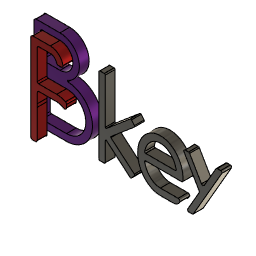
bfkey (Autodesk Fusion 360 design; units mm, degrees)
Autodesk Fusion 360 part; units mm, degrees
sketch "Sketch1" plane through (0, 0, 0) normal (0, 1, 0) x (1, 0, 0)
  line L0 (10, -10) -> (20, -10)
  line L1 (20, -10) -> (20, -150)
  line L2 (20, -150) -> (10, -150)
  line L3 (10, -150) -> (10, -10)
  circle A0 centre (50, -120) radius 30
  circle A1 centre (59.9048, -50.3504) radius 40.3504
  line L4 (20, -150) -> (50, -150)
  line L5 (20, -10) -> (59.9048, -10)
  constraint horizontal L0
  constraint vertical L1
  constraint horizontal L2
  constraint vertical L3
  constraint tangent L1 A0
  constraint coincident A0 L4.end
  constraint tangent A0 L4
  constraint perpendicular L1 L4
  constraint coincident A1 L5.end
  constraint tangent A1 L5
  constraint perpendicular L1 L5
  constraint tangent A0 A1
extrude "Extrude1" add sketch "Sketch1" along normal blind 15 makes body 1
sketch "Sketch2" plane through (0, 0, 0) normal (0, -1, 0) x (1, 0, 0)
  line L0 (50, 150) -> (10, 150)
  line L1 (10, 150) -> (10, 10)
  line L2 (10, 10) -> (59.9048, 10)
  arc A0 (59.9048, 10) -> (54.2238, 90.2988) centre (59.9048, 50.3504) ccw
  arc A1 (54.2238, 90.2988) -> (50, 150) centre (50, 120) ccw
  circle A2 centre (50, 120) radius 20
  line L3 (20, 140) -> (50, 140)
  line L4 (50, 140) -> (50, 100)
  line L5 (50, 100) -> (20, 100)
  line L6 (20, 100) -> (20, 140)
  circle A3 centre (59.9048, 50.3504) radius 30
  line L7 (60.0309, 20.3506) -> (60.0309, 80.3501)
  line L8 (60.0309, 80.3501) -> (20, 80.3501)
  line L9 (20, 80.3501) -> (20, 20.3506)
  line L10 (20, 20.3506) -> (60.0309, 20.3506)
  dimension "d3" = 60
  constraint concentric A1 A2
  constraint horizontal L3
  constraint vertical L4
  constraint horizontal L5
  constraint vertical L6
  constraint coincident A2 L4.end
  constraint concentric A0 A3
  constraint perpendicular L7 L8
  constraint parallel L7 L9
  constraint parallel L8 L10
  constraint coincident A3 L7.end
  constraint vertical L7
  constraint coincident A3 L7.start
  measures "d3" diameter of A3
extrude "Extrude2" cut sketch "Sketch2" against normal blind 50 contours A2 L4 | A2 L4 | A2 L3 L5 L6 | A3 L7 | L7 L8 L9 L10 bodies 1
sketch "Sketch3" plane through (0, 0, 0) normal (0, -1, 0) x (1, 0, 0)
  line L0 (20, 140) -> (50, 140)
  arc A0 (50, 100) -> (50, 140) centre (50, 120) ccw
  line L1 (50, 100) -> (20, 100)
  line L2 (20, 100) -> (20, 140)
  arc A1 (60.0309, 20.3506) -> (60.0309, 80.3501) centre (59.9048, 50.3504) ccw
  line L3 (60.0309, 20.3506) -> (20, 20.3506)
  line L4 (20, 20.3506) -> (20, 80.3501)
  line L5 (20, 80.3501) -> (60.0309, 80.3501)
  line L6 (50, 150) -> (10, 150)
  line L7 (10, 150) -> (10, 10)
  line L8 (10, 10) -> (59.9048, 10)
  arc A2 (59.9048, 10) -> (54.2238, 90.2988) centre (59.9048, 50.3504) ccw
  arc A3 (54.2238, 90.2988) -> (50, 150) centre (50, 120) ccw
  line L9 (20, 0.7007) -> (30, 0.7007)
  line L10 (30, 0.7007) -> (30, 140)
  line L11 (30, 140) -> (20, 140)
  line L12 (20, 140) -> (20, 0.7007)
  line L13 (30, 130) -> (50, 130)
  line L14 (50, 130) -> (50, 140)
  line L15 (50, 140) -> (30, 140)
  line L16 (30, 140) -> (30, 130)
  circle A4 centre (50, 120) radius 20
  circle A5 centre (50, 120) radius 10
  line L17 (60, 120) -> (70, 120)
  circle A6 centre (59.9048, 50.3504) radius 30
  circle A7 centre (59.9048, 50.3504) radius 20
  line L18 (30, 70.3504) -> (60.0309, 70.3504)
  line L19 (60.0309, 70.3504) -> (60.0309, 80.3501)
  line L20 (60.0309, 80.3501) -> (30, 80.3501)
  line L21 (30, 80.3501) -> (30, 70.3504)
  line L22 (75.1346, 63.3138) -> (75.1346, 79.1838)
  dimension "d6" = 40
  constraint horizontal L9
  constraint vertical L10
  constraint horizontal L11
  constraint vertical L12
  constraint coincident L0 L10.end
  constraint horizontal L13
  constraint vertical L14
  constraint horizontal L15
  constraint vertical L16
  constraint coincident L0.end A0.end
  constraint coincident L10 L13.start
  constraint concentric A0 A4
  constraint concentric A4 A5
  constraint coincident L13.end A5
  constraint coincident A5 L17.start
  constraint midpoint A0 L17.end
  constraint horizontal L17
  constraint concentric A1 A6
  constraint coincident A1.end A6
  constraint concentric A1 A7
  constraint horizontal L18
  constraint vertical L19
  constraint horizontal L20
  constraint vertical L21
  constraint coincident A1.end L5.end
  constraint midpoint L10 L18.start
  constraint coincident A7 L22.start
  constraint vertical L22
  constraint tangent A7 L18
  measures "d6" diameter of A7
extrude "Extrude3" add sketch "Sketch3" along normal blind 15 separate body contours A6 L18 L19 | L0 L1 L2 L10 L11 L12 L16 | L0 L10 L13 L15 L16 A4 | L1 L5 L10 L12 | A0 L14 A4 A5 L17 | L13 L14 A4 | L3 L4 L5 L10 L12 A6 L21 | A1 A6 A7 L19 L22 | L5 L10 A6 L18 L20 L21 | L3 L8 L10 L12 | L8 L9 L10 L12 makes body 2
fillet "Fillet1" radius 3 2 edges at (75.1346, -7.5, 63.3138) (60, -7.5, 120) on bodies 2
fillet "Fillet2" radius 3 2 edges at (70, -7.5, 120) (75.1346, -7.5, 76.1971) on bodies 2
fillet "Fillet3" radius 3 5 edges at (10, 7.5, 10) (10, 7.5, 150) (20, -7.5, 0.7007) (30, -7.5, 0.7007) (20, -7.5, 140) on bodies 1 2
fillet "Fillet4" radius 1 1 edges at (54.2238, 7.5, 90.2988) on bodies 1
fillet "Fillet5" radius 2 7 edges at (20, 7.5, 100) (20, 7.5, 20.3506) (20, 7.5, 140) (20, 7.5, 80.3501) (30, -7.5, 70.3504) (30, -7.5, 130) (30, -7.5, 80.3501) on bodies 1 2
sketch "Sketch4" plane through (0, 0, 0) normal (0, 1, 0) x (1, 0, 0)
  line L0 (111.5, -130) -> (118.5, -130)
  line L1 (120, -128.5) -> (120, -11.5)
  line L2 (118.5, -10) -> (111.5, -10)
  line L3 (110, -11.5) -> (110, -128.5)
  line L4 (120, -56.5548) -> (158.3094, -89.03)
  line L5 (160.4235, -88.8558) -> (164.95, -83.5162)
  line L6 (164.7757, -81.402) -> (120, -43.4452)
  line L7 (120, -43.4452) -> (158.3094, -10.97)
  line L8 (160.4235, -11.1442) -> (164.95, -16.4838)
  line L9 (120, -56.5548) -> (164.7757, -18.598)
  line L10 (35, -90) -> (215, -90)
  line L11 (15, -10) -> (188.2335, -10)
  line L12 (159.4536, -90) -> (159.4536, 37.9614)
  arc A0 (158.3094, -89.03) -> (160.4235, -88.8558) centre (159.2793, -87.8858) ccw
  arc A1 (164.95, -83.5162) -> (164.7757, -81.402) centre (163.8058, -82.5462) ccw
  arc A2 (164.7757, -18.598) -> (164.95, -16.4838) centre (163.8058, -17.4538) ccw
  arc A3 (160.4235, -11.1442) -> (158.3094, -10.97) centre (159.2793, -12.1142) ccw
  arc A4 (120, -11.5) -> (118.5, -10) centre (118.5, -11.5) ccw
  arc A5 (111.5, -10) -> (110, -11.5) centre (111.5, -11.5) ccw
  arc A6 (110, -128.5) -> (111.5, -130) centre (111.5, -128.5) ccw
  arc A7 (118.5, -130) -> (120, -128.5) centre (118.5, -128.5) ccw
  line L13 (90, -90) -> (140, -90)
  point P0 (110, -130)
  point P1 (120, -130)
  point P2 (110, -10)
  point P3 (165.9199, -82.372)
  point P4 (159.4536, -10)
  point P5 (165.9199, -17.628)
  dimension "d19" = 10
  dimension "d20" = 10
  dimension "d21" = 10
  dimension "d22" = 120
  dimension "d23" = 1.5
  constraint horizontal L0
  constraint vertical L1
  constraint horizontal L2
  constraint vertical L3
  constraint coincident L1 L4.start
  constraint perpendicular L4 L5
  constraint coincident L1 L6.end
  constraint perpendicular L5 L6
  constraint perpendicular L7 L8
  constraint parallel L7 L9
  constraint perpendicular L1 L10
  constraint perpendicular L1 L11
  constraint coincident P4 L11
  constraint coincident L12.start L10
  constraint perpendicular L11 L12
  constraint coincident P4 L12
  constraint coincident L12.start L4
  constraint coincident L12.start L5
  constraint tangent L4 A0
  constraint tangent L5 A0
  constraint coincident P3 L6
  constraint coincident P3 L5
  constraint tangent L6 A1
  constraint tangent L5 A1
  constraint equal A0 A1
  constraint coincident P5 L9
  constraint coincident P5 L8
  constraint tangent L9 A2
  constraint tangent L8 A2
  constraint equal A0 A2
  constraint coincident P4 L7
  constraint coincident P4 L8
  constraint tangent L7 A3
  constraint tangent L8 A3
  constraint equal A0 A3
  constraint tangent L1 A4
  constraint tangent L2 A4
  constraint equal A0 A4
  constraint coincident P2 L2
  constraint coincident P2 L3
  constraint tangent L2 A5
  constraint tangent L3 A5
  constraint equal A0 A5
  constraint coincident P0 L0
  constraint tangent L0 A6
  constraint tangent L3 A6
  constraint equal A0 A6
  constraint coincident P1 L0
  constraint coincident P1 L1
  constraint tangent L0 A7
  constraint tangent L1 A7
  constraint equal A0 A7
  constraint horizontal L13
  constraint collinear L10 L13
  measures "d19" distance of L12.start P3
  measures "d20" distance of P4 P5
  measures "d21" distance of P0 P1
  measures "d22" distance of P0 P2
  measures "d23" radius of A0
extrude "Extrude4" add sketch "Sketch4" along normal blind 15 separate body contours L0 L1 L3 L10 A6 A7 L13 | L1 L2 L3 L10 L11 A4 A5 L13 | L4 L6 L9 L12 A0 | L1 L6 L9 | L6 L7 L9 L12 A3 | L5 L6 L12 A0 A1 | L8 L9 L12 A2 A3 makes body 3
fillet "Fillet6" radius 1 3 edges at (120, 7.5, 56.5548) (127.7324, 7.5, 50) (120, 7.5, 43.4452) on bodies 3
sketch "Sketch5" plane through (0, 0, 0) normal (0, 1, 0) x (1, 0, 0)
  line L0 (130, -90) -> (325.0868, -90)
  line L1 (130, -10) -> (402.8114, -10)
  line L2 (165.0121, -82.571) -> (165.0121, -120)
  ellipse E0 centre (205.0121, -50) end of major axis (205.0121, -90) minor radius 35
  line L3 (205.0121, -10) -> (205.0121, -90)
  line L4 (170.0121, -50) -> (240.0121, -50)
  ellipse E1 centre (205.0121, -50) end of major axis (205.0121, -80) minor radius 25
  line L5 (205.0121, -20) -> (205.0121, -80)
  line L6 (180.0121, -50) -> (230.0121, -50)
  line L7 (169.0049, -55) -> (248.0049, -55)
  line L8 (167.7908, -45) -> (247.7908, -45)
  line L9 (205.0121, -20) -> (235.2836, -20)
  line L10 (235.2836, -20) -> (235.2836, -10)
  line L11 (205.0121, -10) -> (235.2836, -10)
  line L12 (240.0121, -50) -> (240.0121, -128.7353)
  dimension "d28" = 35
  dimension "d29" = 40
  dimension "d30" = 25
  dimension "d31" = 30
  dimension "d47" = 40
  dimension "d48" = 10
  dimension "d49" = 5
  constraint horizontal L0
  constraint horizontal L1
  constraint perpendicular L0 L2
  constraint perpendicular L0 L3
  constraint coincident E0 L3.start
  constraint coincident E0 L3.end
  constraint coincident E0 L4.start
  constraint coincident E0 L4.end
  constraint concentric E0 E1
  constraint perpendicular L0 L5
  constraint coincident E1 L5.start
  constraint coincident E1 L5.end
  constraint coincident E1 L6.start
  constraint coincident E1 L6.end
  constraint perpendicular L5 L7
  constraint horizontal L8
  constraint perpendicular L3 L9
  constraint coincident L1 L10.end
  constraint perpendicular L1 L10
  constraint perpendicular L0 L12
  measures "d29" distance of E0
  measures "d31" distance of E1
  measures "d47" distance of L2 L5
  measures "d48" distance of L7 L8
  measures "d49" distance of L4 L7
extrude "Extrude5" add sketch "Sketch5" along normal blind 15 separate body contours E0 L3 E1 L7 | E0 L3 E1 L7 | E0 L4 E1 L7 | E0 L4 E1 L7 | E0 L4 E1 L8 | L3 L4 E1 L5 L6 L7 | E0 L4 E1 L8 | L3 L4 E1 L5 L6 L7 | L3 L4 E1 L5 L6 L8 | E0 L3 E1 L8 | L3 L4 E1 L5 L6 L8 | E0 L3 L9 | L1 E0 L9 L10 L11 makes body 4
fillet "Fillet8" radius 1.5 3 edges at (180.3617, 7.5, 55) (229.6624, 7.5, 55) (180.3617, 7.5, 45) on bodies 4
fillet "Fillet9" radius 1.5 1 edges at (239.7376, 7.5, 45) on bodies 4
sketch "Sketch6" plane through (0, 0, 0) normal (0, 1, 0) x (1, 0, 0)
  line L0 (160, -90) -> (455, -90)
  line L1 (210, -10) -> (430, -10)
  line L2 (255.325, -10) -> (301.513, -90)
  line L3 (245.325, -10) -> (291.513, -90)
  line L4 (291.513, -90) -> (301.513, -90)
  line L5 (275.5323, -45) -> (249.5515, -90)
  line L6 (275.5323, -45) -> (346.9943, -45) construction
  line L7 (200, -55) -> (201.1422, -55)
  line L8 (201.1422, -55) -> (371.9878, -55)
  line L9 (205, -45) -> (380, -45)
  line L10 (265.5323, -45) -> (239.5515, -90)
  line L11 (229.5515, -49.5825) -> (229.5515, -112.4125)
  line L12 (239.5515, -90) -> (239.5515, -10)
  dimension "d40" = 60
  dimension "d41" = 10
  dimension "d42" = 120
  dimension "d46" = 10
  constraint horizontal L0
  constraint horizontal L1
  constraint coincident L1 L2.start
  constraint coincident L0 L2.end
  constraint coincident L1 L3.start
  constraint coincident L0 L3.end
  constraint parallel L2 L3
  constraint horizontal L6
  constraint coincident L2 L5.start
  constraint coincident L0 L5.end
  constraint horizontal L7
  constraint parallel L7 L8
  constraint horizontal L9
  constraint coincident L5.start L9
  constraint coincident L3 L10.start
  constraint coincident L9 L10.start
  constraint parallel L5 L10
  constraint perpendicular L0 L11
  constraint perpendicular L1 L12
  constraint coincident L0 L10.end
  constraint coincident L12 L10.end
  measures "d40" angle of L1 L2
  measures "d41" distance of L2.end L3.end
  measures "d42" angle of L5 L6
  measures "d46" distance of L11 L12
extrude "Extrude6" add sketch "Sketch6" along normal blind 15 separate body contours L0 L5 L8 L10 | L3 L5 L8 L10 | L0 L2 L3 L4 L8 | L3 L5 L8 | L3 L5 L9 | L1 L2 L3 L9 | L2 L3 L5 L8 makes body 5
fillet "Fillet10" radius 3 1 edges at (235.2836, 7.5, 20) on bodies 4
fillet "Fillet11" radius 11 1 edges at (235.2836, 7.5, 10) on bodies 4
fillet "Fillet12" radius 2 6 edges at (239.5515, 7.5, 90) (249.5515, 7.5, 90) (291.513, 7.5, 90) (301.513, 7.5, 90) (245.325, 7.5, 10) (255.325, 7.5, 10) on bodies 5
fillet "Fillet13" radius 3 1 edges at (265.5323, 7.5, 45) on bodies 5
fillet "Fillet14" radius 2.5 2 edges at (269.7588, 7.5, 55) (271.3058, 7.5, 55) on bodies 5
